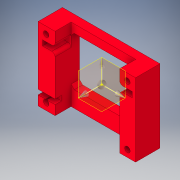
# Autodesk Inventor part: EDMO1-1_Cover
Saved by Autodesk Inventor 2019 (Build 230136000, 136)
## iProperties
Created: 2016-10-24
Part Number: EDMO1-1_Cover
Material: PLA
Document SubType Name: Modeling
Designer: Lucas
Density: 1.29985 g/cm^3
Appearance: Plastic Vinyl
Mass: 22.8661 g
Surface Area: 95.8167 cm^2
Volume: 17.5914 cm^3
Author: Lucas
Autodesk Inventor part; units mm, degrees
ref_plane "YZ Plane" through (0, 0, 0) normal (1, 0, 0) x (0, 1, 0)
ref_plane "XZ Plane" through (0, 0, 0) normal (0, 1, 0) x (-1, 0, 0)
ref_plane "XY Plane" through (0, 0, 0) normal (0, 0, 1) x (1, 0, 0)
sketch "Sketch2" plane through (0, 0, 0) normal (0, 0, 1) x (1, 0, 0)
  line L0 (0, 0) -> (60, 0)
  line L1 (60, 0) -> (60, 45)
  line L2 (60, 45) -> (0, 45)
  line L3 (0, 45) -> (0, 0)
  dimension "d0" = 60
  dimension "d1" = 45
  constraints: 8 end point, 2 parallel, 1 horizontal, 1 perpendicular
  measures "d0" distance of L2.end L1.end
  measures "d1" distance of L1.end L0.end
extrude "Cover_Body" add sketch "Sketch2" along normal blind 15
sketch "Sketch4" plane through (0, 0, 15) normal (0, 0, 1) x (1, 0, 0)
  line L0 (60, 45) -> (0, 45) projected
  line L1 (0, 45) -> (0, 0) projected
  line L2 (2.75, 33.35) -> (10.45, 33.35)
  line L3 (50.25, 33.35) -> (57.95, 33.35)
  line L4 (60, 0) -> (60, 45) projected
  line L5 (0, 0) -> (60, 0) projected
  line L6 (2.75, 33.35) -> (2.75, 36.65)
  line L7 (2.75, 36.65) -> (10.45, 36.65)
  line L8 (10.45, 36.65) -> (10.45, 45)
  line L9 (57.95, 36.65) -> (57.95, 33.35)
  line L10 (57.95, 36.65) -> (50.25, 36.65)
  line L11 (50.25, 36.65) -> (50.25, 45)
  line L12 (10.45, 45) -> (50.25, 45)
  line L13 (30, 36.5125) -> (30, -47.625) construction
  line L14 (50.25, 33.35) -> (50.25, 0)
  line L15 (10.45, 33.35) -> (10.45, 0)
  line L16 (10.45, 0) -> (50.25, 0)
  line L17 (-12.9814, 35) -> (83.563, 35) construction
  dimension "d6" = 7.7
  dimension "d14" = 3.3
  dimension "d15" = 3.3
  dimension "d22" = 60
  dimension "d23" = 30
  dimension "d28" = 7.7
  dimension "d118" = 39.8
  dimension "d130" = 33.35
  dimension "d140" = 36.65
  dimension "d141" = 10
  dimension "d142" = 10.45
  constraints: 28 end point, 6 collinear, 4 perpendicular, 4 point on line, 3 horizontal, 2 vertical, 1 other
  measures "d6" distance of L2.start L2.end
  measures "d14" distance of L2.start L6.end
  measures "d15" distance of L9.start L3.end
  measures "d22" distance between parallel lines of L4 L1
  measures "d23" distance between parallel lines of L13 L1
  measures "d28" distance of L9.start L10.end
  measures "d118" distance between parallel lines of L15 L14
  measures "d130" distance of L2.end L15.end
  measures "d140" distance between parallel lines of L5 L7
  measures "d141" distance between parallel lines of L0 L17
  measures "d142" distance between parallel lines of L15 L1
extrude "Servo_Intake" cut sketch "Sketch4" against normal blind 9.85 contours L11 L10 L9 L3 L14 L5 L15 L2 L6 L7 L8 L0
sketch "Sketch5" plane through (0, 0, 15) normal (0, 0, 1) x (1, 0, 0)
  line L0 (0, 5.9) -> (0, 8.9)
  line L1 (-28.5301, 7.4) -> (55.9395, 7.4) construction
  line L2 (0, 8.9) -> (10.45, 8.9)
  line L3 (10.45, 8.9) -> (10.45, 5.9)
  line L4 (10.45, 5.9) -> (0, 5.9)
  line L5 (10.45, 0) -> (10.45, 33.35) projected
  line L6 (0, 45) -> (0, 0) projected
  line L7 (0, 0) -> (10.45, 0) projected
  dimension "d97" = 3
  dimension "d137" = 5.9
  dimension "d153" = 7.4
  constraints: 10 end point, 2 collinear, 2 horizontal, 1 other
  measures "d97" distance of L2.end L3.end
  measures "d137" distance between parallel lines of L4 L7
  measures "d153" distance between parallel lines of L7 L1
extrude "Cable_Opening" cut sketch "Sketch5" against normal blind 4 contours L0 L2 L3 L4
sketch "Sketch6" plane through (0, 0, 15) normal (0, 0, 1) x (1, 0, 0)
  circle A0 centre (5, 40.75) radius 1.7
  circle A1 centre (55, 40.75) radius 1.7
  circle A2 centre (55, 4.25) radius 1.7
  circle A3 centre (5, 4.25) radius 1.7
  line L0 (30, 47.1) -> (30, -0.525) construction
  line L1 (-11.6375, 22.5) -> (75.675, 22.5) construction
  line L2 (60, 0) -> (60, 45) projected
  line L3 (0, 45) -> (0, 0) projected
  line L4 (10.45, 45) -> (0, 45) projected
  line L5 (0, 0) -> (60, 0) projected
  point P0 (42, 12.35)
  point P1 (0, 12.35)
  dimension "d29" = 3.4
  dimension "d30" = 3.4
  dimension "d31" = 3.4
  dimension "d32" = 3.4
  dimension "d33" = 60
  dimension "d34" = 30
  dimension "d35" = 45
  dimension "d36" = 22.5
  dimension "d37" = 50
  dimension "d38" = 25
  dimension "d39" = 36.5
  dimension "d40" = 18.25
  constraints: 4 centre point, 4 end point, 2 horizontal alignment, 2 vertical alignment, 1 horizontal, 1 other
  measures "d29" diameter of A0
  measures "d30" diameter of A1
  measures "d31" diameter of A2
  measures "d32" diameter of A3
  measures "d34" distance between parallel lines of L0 L3
  measures "d35" distance between parallel lines of L4 L5
  measures "d36" distance between parallel lines of L4 L1
  measures "d37" distance of A1.centre A0.centre
  measures "d38" distance from line of L0 A0.centre
  measures "d39" distance of A3.centre A0.centre
  measures "d40" distance from line of L1 A2.centre
extrude "Screw_Holes" cut sketch "Sketch6" against normal blind 36.5
sketch "Sketch16" plane through (0, 0, 0) normal (0, 0, -1) x (-1, 0, 0)
  circle A0 centre (-55, 4.25) radius 3.25
  circle A1 centre (-5, 40.75) radius 3.25
  circle A2 centre (-55, 4.25) radius 1.7 projected
  circle A3 centre (-5, 40.75) radius 1.7 projected
  circle A4 centre (-5, 4.25) radius 1.7 projected
  circle A5 centre (-5, 4.25) radius 3.25
  circle A6 centre (-55, 40.75) radius 1.7 projected
  circle A7 centre (-55, 40.75) radius 3.25
  dimension "d99" = 6.5
  dimension "d100" = 6.5
  dimension "d151" = 6.5
  dimension "d152" = 6.5
  constraints: 4 centre point, 2 coincident, 2 concentric
  measures "d99" diameter of A0
  measures "d100" diameter of A1
  measures "d151" diameter of A5
  measures "d152" diameter of A7
extrude "Screw_Pockets" cut sketch "Sketch16" against normal blind 9 contours A0 | A1 | A2 | A3 | A5 | A7
sketch "Sketch24" plane through (0, 0, 5.15) normal (0, 0, 1) x (1, 0, 0)
  line L0 (10.45, 9.9) -> (50.25, 9.9)
  line L1 (50.25, 9.9) -> (50.25, 40)
  line L2 (50.25, 40) -> (10.45, 40)
  line L3 (10.45, 40) -> (10.45, 9.9)
  line L4 (50.25, 0) -> (10.45, 0) projected
  line L5 (10.45, 45) -> (50.25, 45) projected
  line L6 (10.45, 0) -> (10.45, 33.35) projected
  line L7 (50.25, 33.35) -> (50.25, 0) projected
  point P0 (0, 0)
  dimension "d143" = 9.9
  dimension "d144" = 5
  constraints: 8 end point, 2 collinear, 2 parallel, 1 horizontal, 1 perpendicular
  measures "d143" distance between parallel lines of L0 L4
  measures "d144" distance between parallel lines of L5 L2
extrude "Cooling_Opening" cut sketch "Sketch24" against normal up to surface (5.15 mm away) contours L3 L2 L1 L0
chamfer "Chamfer1" distance 2 angle 45 4 edges at (10.45, 9.9, 2.575) (50.25, 9.9, 2.575) (50.25, 40, 2.575) (10.45, 40, 2.575)
fillet "Fillet2" radius 2 4 edges at (10.45, 36.65, 10.075) (10.45, 33.35, 10.075) (50.25, 36.65, 10.075) (50.25, 33.35, 10.075)
equation "\"d15\" = d14"
equation "\"d23\" = 0.5 * d22"
equation "\"d28\" = d6"
equation "\"d30\" = d29"
equation "\"d31\" = d29"
equation "\"d32\" = d29"
equation "\"d34\" = 0.5 * d33"
equation "\"d36\" = 0.5 * d35"
equation "\"d38\" = 0.5 * d37"
equation "\"d40\" = 0.5 * d39"
equation "\"d41\" = d39"
equation "\"d99\" = d100"
equation "\"d151\" = d100"
equation "\"d152\" = d100"
body "Solid1"
